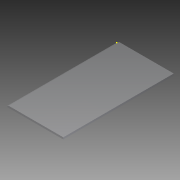
# Autodesk Inventor part: teto01
Saved by Autodesk Inventor 2015 (Build 190159000, 159)
## iProperties
Created: 2016-08-07
Part Number: teto01
Material: Polycarbonate, Clear
Document SubType Name: Modeling
Designer: Gabriel
Density: 1.2 g/cm^3
Appearance: Polycarbonate - Clear
Author: Gabriel
Autodesk Inventor part; units mm, degrees
ref_plane "YZ Plane" through (0, 0, 0) normal (1, 0, 0) x (0, 1, 0)
ref_plane "XZ Plane" through (0, 0, 0) normal (0, 1, 0) x (-1, 0, 0)
ref_plane "XY Plane" through (0, 0, 0) normal (0, 0, 1) x (1, 0, 0)
sketch "Sketch1" plane through (0, 0, 0) normal (0, 0, 1) x (1, 0, 0)
  point P0 (0, 0)
sketch "Sketch2" plane through (0, 0, 0) normal (0, 0, 1) x (1, 0, 0)
  line L0 (0, 0) -> (219, 0)
  line L1 (219, 0) -> (219, 7)
  line L2 (219, 7) -> (0, 7)
  line L3 (0, 7) -> (0, 0)
  dimension "d0" = 219
  dimension "d1" = 7
  constraints: 8 end point, 2 parallel, 1 horizontal, 1 perpendicular
  measures "d0" distance of L2.end L1.end
  measures "d1" distance of L1.end L0.end
extrude "Extrusion1" add sketch "Sketch2" along normal blind 424
sketch "Sketch4" plane through (0, 0, 0) normal (0, 0, -1) x (-1, 0, 0)
  line L0 (0, 0) -> (15.4114, 0)
  line L1 (0, 0) -> (12.5833, -9.3896)
  line L2 (0, 0) -> (15.7004, 0) construction
  line L3 (0, 0) -> (-16.5192, 12.3265)
  line L4 (-219, 7) -> (0, 7) projected
  line L5 (-9.381, 7) -> (0, 7)
  line L6 (0, 7) -> (0, 0)
  dimension "d7" = 36.73
  constraints: 12 end point, 3 point on line, 2 horizontal, 1 collinear, 1 equal length, 1 perpendicular
  measures "d7" angle of L1 L2
extrude "Extrusion3" cut sketch "Sketch4" against normal blind 577.375
body "Solid1"
